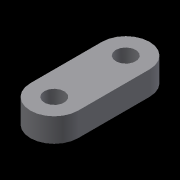
# Autodesk Inventor part: VibroMount
Saved by Autodesk Inventor 2015 SP1 (Build 190203100, 203)
## iProperties
Created: 2015-07-23
Part Number: VibroMount
Material: Generic
Document SubType Name: Modeling
Designer: Val
Density: 1 g/cm^3
Appearance: Default
Author: Val
Autodesk Inventor part; units mm, degrees
ref_plane "YZ Plane" through (0, 0, 0) normal (1, 0, 0) x (0, 1, 0)
ref_plane "XZ Plane" through (0, 0, 0) normal (0, 1, 0) x (-1, 0, 0)
ref_plane "XY Plane" through (0, 0, 0) normal (0, 0, 1) x (1, 0, 0)
sketch "Base" plane through (0, 0, 0) normal (0, 0, 1) x (1, 0, 0)
  circle A0 centre (0, 0) radius 3
  line L0 (0, 0) -> (0, -9) construction
  circle A1 centre (0, -9) radius 3
  line L1 (-3, 0) -> (-3, -9)
  line L2 (3, -9) -> (3, 0)
  dimension "d0" = 6
  dimension "d1" = 9
  constraints: 6 end point, 4 point on circle, 4 tangent, 2 centre point, 2 coincident, 1 equal radius, 1 vertical
  measures "d0" diameter of A0
  measures "d1" distance of L0.start L0.end
extrude "BaseFeature" add sketch "Base" along normal blind 3
hole "MountHolesFeature" at (0, 0, 0) at (0, -9, 0) at (0, -9, 0) direction (0, 0, 1) diameter 2.5 end through all
